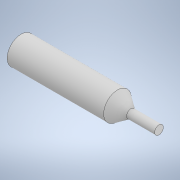
# Autodesk Inventor part: nozzle mould tool kndx
Saved by Autodesk Inventor 2021 (Build 250183000, 183)
## iProperties
Created: 2021-04-27
Part Number: nozzle mould tool kndx
Material: Generic
Document SubType Name: Modeling
Designer: samlo
Density: 1 g/cm^3
Appearance: Default
Author: samlo
Autodesk Inventor part; units mm, degrees
ref_plane "YZ Plane" through (0, 0, 0) normal (1, 0, 0) x (0, 1, 0)
ref_plane "XZ Plane" through (0, 0, 0) normal (0, 1, 0) x (-1, 0, 0)
ref_plane "XY Plane" through (0, 0, 0) normal (0, 0, 1) x (1, 0, 0)
sketch "Sketch1" plane through (0, 0, 0) normal (0, 0, 1) x (1, 0, 0)
  line L0 (0, 0) -> (150, 0)
  line L1 (150, 0) -> (150, 4.75)
  line L2 (150, 4.75) -> (119.4815, 4.75)
  line L3 (119.4815, 4.75) -> (104.843, 15)
  line L4 (104.843, 15) -> (0, 15)
  line L5 (0, 15) -> (0, 0)
  dimension "d0" = 15
  dimension "d1" = 4.75
  dimension "d3" = 45.157
  dimension "d4" = 125
  dimension "d5" = 150
  constraints: 12 end point, 2 perpendicular, 1 horizontal, 1 parallel, 1 vertical
  measures "d0" distance of L4.end L0.start
  measures "d1" distance of L0.end L1.end
  measures "d3" horizontal distance of L0.end L3.end
  measures "d4" angle of L5 L3
  measures "d5" distance of L0.start L0.end
revolve "Revolution1" add sketch "Sketch1" angle 360 about axis through (0, 0, 0) along (1, 0, 0)
body "Solid1"
